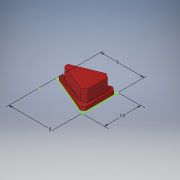
# Autodesk Inventor part: SideButton
Saved by Autodesk Inventor 2019 (Build 230136000, 136)
## iProperties
Created: 2021-04-22
Part Number: SideButton
Material: Všeobecné
Document SubType Name: Modeling
Designer: miko flosso
Density: 1 g/cm^3
Appearance: Červená
Author: miko flosso
Autodesk Inventor part; units mm, degrees
ref_plane "YZ Plane" through (0, 0, 0) normal (1, 0, 0) x (0, 1, 0)
ref_plane "XZ Plane" through (0, 0, 0) normal (0, 1, 0) x (-1, 0, 0)
ref_plane "XY Plane" through (0, 0, 0) normal (0, 0, 1) x (1, 0, 0)
sketch "Náčrt1" plane through (0, 0, 0) normal (0, 1, 0) x (-1, 0, 0)
  line L0 (-9, 0.0297) -> (-9, -7.4703)
  line L1 (-9, -7.4703) -> (0, -3.75)
  line L2 (-9, 0.0297) -> (0, -3.75)
  point P0 (0, 0)
  dimension "d1" = 7.5
  dimension "d21" = 9
  dimension "d22" = 9
  constraints: 6 end point
  measures "d1" distance of L0.end L0.start
  measures "d21" horizontal distance of L0.end L1.end
  measures "d22" horizontal distance of L0.start L1.end
extrude "Vysunutí1" add sketch "Náčrt1" along normal blind 0.8
sketch "Náčrt2" plane through (0, 0.8, 0) normal (0, 1, 0) x (1, 0, 0)
  line L0 (8.5, 0.7703) -> (8.5, 6.6703)
  line L1 (9, -0.0297) -> (9, 7.4703) projected
  line L2 (8.5, 6.6703) -> (1.2, 3.7203)
  line L3 (8.5, 0.7703) -> (1.2, 3.7203)
  point P0 (0, 0)
  dimension "d6" = 0.5
  dimension "d16" = 5.9
  dimension "d17" = 0.8
  dimension "d18" = 2.95
  dimension "d19" = 7.3
  constraints: 6 end point
  measures "d6" distance between parallel lines of L0 L1
  measures "d16" distance of L0.start L0.end
  measures "d17" vertical distance of L1.start L0.start
  measures "d18" vertical distance of L0.end L2.end
  measures "d19" distance from line of L0 L2.end
extrude "Vysunutí2" add sketch "Náčrt2" along normal blind 2.5
chamfer "Zkosení1" distance 0.9 angle 45 3 edges at (1.2, 2.05, -3.7203) (8.5, 2.05, -0.7703) (8.5, 2.05, -6.6703)
chamfer "Zkosení2" distance 0.9 angle 45 3 edges at (9, 0.4, 0.0297) (9, 0.4, -7.4703) (0, 0.4, -3.75)
